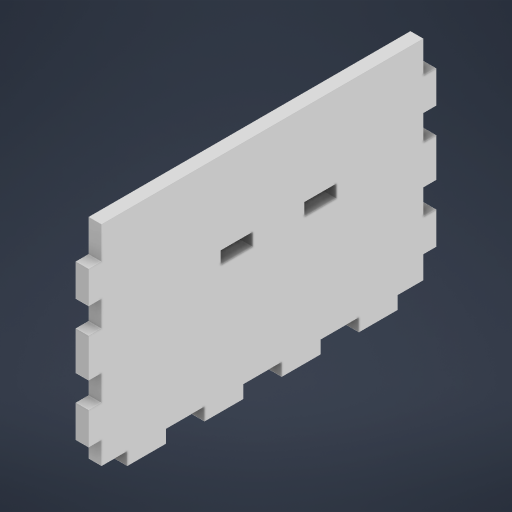
# Autodesk Inventor part: Langbektang houder
Saved by Autodesk Inventor 2023.2 (Build 272271000, 271)
## iProperties
Created: 2020-09-09
Part Number: Langbektang houder
Material: Generic
Document SubType Name: Modeling
Designer: nathan.bollaert
Density: 1 g/cm^3
Appearance: Default
Author: nathan.bollaert
Autodesk Inventor part; units mm, degrees
ref_plane "YZ Plane" through (0, 0, 0) normal (1, 0, 0) x (0, 1, 0)
ref_plane "XZ Plane" through (0, 0, 0) normal (0, 1, 0) x (-1, 0, 0)
ref_plane "XY Plane" through (0, 0, 0) normal (0, 0, 1) x (1, 0, 0)
sketch "Sketch1" plane through (0, 0, 0) normal (1, 0, 0) x (0, 1, 0)
  line L0 (0, 0) -> (69, 0)
  line L1 (69, 0) -> (69, -108)
  line L2 (69, -108) -> (0, -108)
  line L3 (0, -108) -> (0, 0)
  dimension "d228" = 69
  dimension "d229" = 108
  constraints: 8 end point, 2 parallel, 1 horizontal, 1 perpendicular
  measures "d228" distance of L1.end L2.end
  measures "d229" distance of L0.end L1.end
extrude "Extrusion1" add sketch "Sketch1" against normal blind 4
sketch "Sketch2" plane through (0, 0, 0) normal (1, 0, 0) x (0, 0, -1)
  line L0 (54, 69) -> (54, 0)
  line L1 (108, 0) -> (0, 0) projected
  line L2 (0, 0) -> (0, 69) projected
  line L3 (0, 34.5) -> (108, 34.5)
  line L4 (108, 69) -> (108, 0) projected
  line L5 (0, 0) -> (108, 0)
  line L6 (12, 0) -> (12, 4)
  line L7 (4, 0) -> (12, 0)
  line L8 (4, 59) -> (4, 49)
  line L9 (4, 49) -> (0, 49)
  line L10 (0, 49) -> (0, 41)
  line L11 (0, 41) -> (4, 41)
  line L12 (4, 41) -> (4, 29)
  line L13 (4, 29) -> (0, 29)
  line L14 (0, 29) -> (0, 21)
  line L15 (0, 21) -> (4, 21)
  line L16 (4, 21) -> (4, 11)
  line L17 (4, 11) -> (0, 11)
  line L18 (0, 69) -> (0, 0) projected
  line L19 (108, 0) -> (108, 69)
  line L20 (108, 34.5) -> (0, 34.5)
  line L21 (108, 49) -> (108, 41)
  line L22 (108, 29) -> (108, 21)
  line L23 (108, 69) -> (108, 0)
  line L24 (4, 59) -> (0, 59)
  line L25 (0, 0) -> (108, 0) projected
  line L26 (108, 69) -> (0, 69) projected
  line L27 (108, 0) -> (108, 69)
  line L28 (108, 34.5) -> (0, 34.5)
  line L29 (104, 59) -> (104, 49)
  line L30 (104, 49) -> (108, 49)
  line L31 (108, 49) -> (108, 41)
  line L32 (108, 41) -> (104, 41)
  line L33 (104, 41) -> (104, 29)
  line L34 (104, 29) -> (108, 29)
  line L35 (108, 29) -> (108, 21)
  line L36 (108, 21) -> (104, 21)
  line L37 (104, 21) -> (104, 11)
  line L38 (104, 11) -> (108, 11)
  line L39 (108, 69) -> (108, 0)
  line L40 (0, 34.5) -> (108, 34.5)
  line L41 (104, 59) -> (108, 59)
  line L42 (4, 49) -> (4, 41)
  line L43 (4, 29) -> (4, 21)
  line L44 (4, 59) -> (4, 69)
  line L45 (0, 69) -> (108, 69) projected
  line L46 (104, 69) -> (104, 59)
  line L47 (104, 49) -> (104, 41)
  line L48 (104, 29) -> (104, 21)
  line L49 (12, 0) -> (24, 0)
  line L50 (24, 0) -> (24, 4)
  line L51 (24, 4) -> (36, 4)
  line L52 (36, 4) -> (36, 0)
  line L53 (36, 0) -> (24, 0)
  line L54 (36, 0) -> (48, 0)
  line L55 (60, 0) -> (48, 0)
  line L56 (60, 0) -> (72, 0)
  line L57 (72, 0) -> (72, 4)
  line L58 (72, 4) -> (84, 4)
  line L59 (84, 4) -> (84, 0)
  line L60 (84, 0) -> (72, 0)
  line L61 (12, 4) -> (0, 4)
  line L62 (4, 11) -> (4, 0)
  line L63 (104, 11) -> (104, 0)
  line L64 (106, 0) -> (96, 0)
  line L65 (84, 0) -> (96, 0)
  line L66 (48, 0) -> (60, 0)
  line L67 (60, 0) -> (72, 0)
  line L68 (96, 0) -> (106, 0)
  line L69 (108, 4) -> (108, 11)
  line L70 (60, 0) -> (60, 4)
  line L71 (48, 4) -> (48, 0)
  line L72 (60, 4) -> (48, 4)
  line L73 (96, 4) -> (108, 4)
  line L74 (96, 4) -> (96, 0)
  line L75 (108, 0) -> (108, 69) projected
  line L76 (108, 4) -> (108, 0)
  point P0 (12, 0)
  point P1 (108, 29)
  point P2 (108, 41)
  point P3 (108, 49)
  point P4 (108, 59)
  point P5 (108, 11)
  point P6 (108, 21)
  point P7 (84, 0)
  point P8 (104, 0)
  point P9 (36, 0)
  point P10 (4, 4)
  point P11 (104, 4)
  dimension "d246" = 12
  dimension "d248" = 10
  dimension "d250" = 8
  dimension "d253" = 4
  dimension "d256" = 10
  dimension "d257" = 12
  dimension "d259" = 12
  constraints: 135 end point, 18 symmetric about line, 17 equal length, 16 perpendicular, 16 point on line, 9 collinear, 9 horizontal, 6 vertical, 2 midpoint, 25 other
  measures "d246" distance of L10.end L13.end
  measures "d248" distance of L9.end L24.end
  measures "d250" distance of L9.end L10.end
  measures "d253" distance from line of L5 L61.end
  measures "d256" distance from line of L26 L24.end
  measures "d257" distance of L1.end L6.start
  measures "d259" distance of L6.start L49.end
extrude "Extrusion2" cut sketch "Sketch2" against normal blind 4 contours L26 L4 L41 L46 | L44 L24 L2 L26 | L72 L70 L1 L0 | L0 L1 L71 L72 | L11 L2 L9 L42 | L43 L15 L2 L13 | L47 L30 L4 L32 | L34 L4 L36 L48 | L57 L58 L59 L1 | L1 L50 L51 L52 | L62 L61 L2 L17 | L38 L4 L73 L63 | L62 L1 L2 L61 | L61 L6 L1 L62 | L73 L4 L1 L63 | L63 L1 L74 L73
sketch "Sketch3" plane through (0, 0, 0) normal (1, 0, 0) x (0, 0, -1)
  line L0 (41, 39.5) -> (77, 39.5)
  line L1 (77, 39.5) -> (77, 43.5)
  line L2 (77, 43.5) -> (41, 43.5)
  line L3 (41, 43.5) -> (41, 39.5)
  line L4 (48, 4) -> (60, 4) projected
  line L5 (67, 43.5) -> (67, 39.5)
  line L6 (104, 69) -> (4, 69) projected
  line L7 (54, 69) -> (54, 4)
  line L8 (60, 4) -> (48, 4) projected
  line L9 (51, 43.5) -> (51, 39.5)
  point P0 (0, 0)
  dimension "d264" = 4
  dimension "d265" = 35.5
  dimension "d266" = 26
  dimension "d267" = 10
  dimension "d269" = 10
  constraints: 14 end point, 4 point on line, 3 perpendicular, 2 midpoint, 2 parallel, 1 horizontal, 1 other
  measures "d264" distance of L1.end L0.end
  measures "d265" distance between parallel lines of L4 L0
  measures "d266" distance between parallel lines of L5 L3
  measures "d267" distance between parallel lines of L3 L9
  measures "d269" distance between parallel lines of L1 L5
extrude "Extrusion3" cut sketch "Sketch3" against normal blind 4 contours L3 L2 L9 L0 | L5 L2 L1 L0
body "Solid5"
